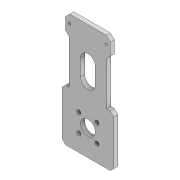
# Autodesk Inventor part: Part1_Camera
Saved by Autodesk Inventor 2021 (Build 250183000, 183)
## iProperties
Created: 2022-06-14
Part Number: Part1_Camera
Material: Generic
Document SubType Name: Modeling
Designer: romanp
Density: 1 g/cm^3
Appearance: Default
Author: romanp
Autodesk Inventor part; units mm, degrees
ref_plane "YZ Plane" through (0, 0, 0) normal (1, 0, 0) x (0, 1, 0)
ref_plane "XZ Plane" through (0, 0, 0) normal (0, 1, 0) x (-1, 0, 0)
ref_plane "XY Plane" through (0, 0, 0) normal (0, 0, 1) x (1, 0, 0)
sketch "Sketch1" plane through (0, 0, 0) normal (0, 0, 1) x (1, 0, 0)
  line L0 (0, 0) -> (54.9443, 0)
  line L1 (54.9443, 0) -> (59.3561, 4.4119)
  line L2 (59.3561, 4.4119) -> (59.3561, 59.3561)
  line L3 (59.3561, 59.3561) -> (54.9443, 63.768)
  line L4 (54.9443, 63.768) -> (0, 63.768)
  line L5 (0, 63.768) -> (-4.4114, 59.3566)
  line L6 (-4.4114, 59.3566) -> (-4.4114, 4.4114)
  line L7 (-4.4114, 4.4114) -> (0, 0)
  circle A0 centre (38.6091, 43.0209) radius 2.5
  circle A1 centre (16.3352, 43.0209) radius 2.5
  circle A2 centre (38.6091, 20.7471) radius 2.5
  circle A3 centre (16.3352, 20.7471) radius 2.5
  circle A4 centre (4.9721, 131.884) radius 1.5
  circle A5 centre (49.9721, 131.884) radius 1.5
  line L8 (0, 131.884) -> (0, 141.884)
  line L9 (0, 141.884) -> (54.9443, 141.884)
  line L10 (54.9443, 141.884) -> (54.9443, 131.884)
  line L11 (0, 131.884) -> (0, 121.884)
  line L12 (54.9443, 121.884) -> (54.9443, 131.884)
  line L13 (0, 121.884) -> (4.4114, 117.4726)
  line L14 (50.5324, 117.4721) -> (54.9443, 121.884)
  line L15 (4.4114, 117.4726) -> (4.4114, 63.768)
  line L16 (50.5324, 117.4721) -> (50.5324, 63.768)
  dimension "d3" = 3
  dimension "d4" = 3
  dimension "d5" = 10
  dimension "d6" = 10
  constraints: 34 end point, 6 centre point, 4 perpendicular, 2 point on line, 2 vertical
  measures "d3" diameter of A4
  measures "d4" diameter of A5
  measures "d5" distance of L8.start L8.end
  measures "d6" distance of L8.start L11.end
extrude "Extrusion1" add sketch "Sketch1" along normal blind 5
chamfer "Chamfer1" distance 5 angle 45 2 edges at (0, 141.884, 2.5) (54.9443, 141.884, 2.5)
sketch "Sketch2" plane through (0, 0, 5) normal (0, 0, 1) x (1, 0, 0)
  line L0 (49.9443, 141.884) -> (54.9443, 136.884) projected
  line L1 (49.9443, 141.884) -> (5, 141.884) projected
  line L2 (0, 136.884) -> (5, 141.884) projected
  line L3 (0, 136.884) -> (0, 121.884) projected
  line L4 (0, 121.884) -> (4.4114, 117.4726) projected
  line L5 (4.4114, 117.4726) -> (4.4114, 63.768) projected
  line L6 (4.4114, 63.768) -> (0, 63.768) projected
  line L7 (0, 63.768) -> (-4.4114, 59.3566) projected
  line L8 (-4.4114, 59.3566) -> (-4.4114, 4.4114) projected
  line L9 (-4.4114, 4.4114) -> (0, 0) projected
  line L10 (0, 0) -> (54.9443, 0) projected
  line L11 (54.9443, 0) -> (59.3561, 4.4119) projected
  line L12 (59.3561, 4.4119) -> (59.3561, 59.3561) projected
  line L13 (59.3561, 59.3561) -> (54.9443, 63.768) projected
  line L14 (54.9443, 63.768) -> (50.5324, 63.768) projected
  line L15 (50.5324, 63.768) -> (50.5324, 117.4721) projected
  line L16 (50.5324, 117.4721) -> (54.9443, 121.884) projected
  line L17 (54.9443, 121.884) -> (54.9443, 136.884) projected
  circle A0 centre (49.9721, 131.884) radius 1.5 projected
  circle A1 centre (4.9721, 131.884) radius 1.5 projected
  circle A2 centre (38.6091, 20.7471) radius 2.5 projected
  circle A3 centre (38.6091, 43.0209) radius 2.5 projected
  circle A4 centre (16.3352, 43.0209) radius 2.5 projected
  circle A5 centre (16.3352, 20.7471) radius 2.5 projected
  circle A6 centre (27.4721, 31.884) radius 9
  dimension "d12" = 18
  constraints: 1 centre point
  measures "d12" diameter of A6
extrude "Extrusion2" cut sketch "Sketch2" against normal blind 5 contours A6
sketch "Sketch3" plane through (0, 0, 5) normal (0, 0, 1) x (1, 0, 0)
  arc A0 (36.4721, 101.884) -> (18.4721, 101.884) centre (27.4721, 101.884) ccw
  line L0 (18.4721, 101.884) -> (18.4721, 81.884)
  line L1 (36.4721, 101.884) -> (36.4721, 81.884)
  circle A1 centre (27.4721, 31.884) radius 9 projected
  line L2 (27.4721, 71.884) -> (27.4721, 81.884)
  arc A2 (18.4721, 81.884) -> (36.4721, 81.884) centre (27.4721, 81.884) ccw
  point P0 (0, 0)
  dimension "d16" = 18
  dimension "d20" = 10
  dimension "d21" = 18
  constraints: 6 end point, 4 point on circle, 2 centre point, 2 tangent, 2 vertical, 1 coincident
  measures "d16" diameter of A0
  measures "d20" distance of L2.start L2.end
  measures "d21" diameter of A2
extrude "Extrusion3" cut sketch "Sketch3" against normal blind 10 contours L1 A2 L0 A0
sketch "Sketch4" plane through (0, 0, 5) normal (0, 0, 1) x (1, 0, 0)
  circle A0 centre (16.3352, 43.0209) radius 2.5 projected
  circle A1 centre (16.3352, 43.0209) radius 2.55
  circle A2 centre (38.6091, 43.0209) radius 2.5 projected
  circle A3 centre (38.6091, 43.0209) radius 2.55
  circle A4 centre (38.6091, 20.7471) radius 2.5 projected
  circle A5 centre (38.6091, 20.7471) radius 2.55
  circle A6 centre (16.3352, 20.7471) radius 2.5 projected
  circle A7 centre (16.3352, 20.7471) radius 2.55
  circle A8 centre (4.9721, 131.884) radius 1.5 projected
  circle A9 centre (4.9721, 131.884) radius 1.55
  circle A10 centre (49.9721, 131.884) radius 1.5 projected
  circle A11 centre (49.9721, 131.884) radius 1.55
  point P0 (0, 0)
  dimension "d22" = 5.1
  dimension "d23" = 5.1
  dimension "d24" = 5.1
  dimension "d25" = 5.1
  dimension "d26" = 3.1
  dimension "d27" = 3.1
  constraints: 6 centre point, 6 coincident
  measures "d22" diameter of A1
  measures "d23" diameter of A3
  measures "d24" diameter of A5
  measures "d25" diameter of A7
  measures "d26" diameter of A9
  measures "d27" diameter of A11
extrude "Extrusion4" cut sketch "Sketch4" against normal blind 10 contours A0 | A1 | A2 | A3 | A4 | A5 | A6 | A7 | A8 | A9 | A10 | A11
body "Solid1"
